Autodesk Fusion 360 part; units mm, degrees
(part 5 of 7)
  spline S20 degree 5 poles (-19.6631, 0.6054) (-19.6646, 0.6091) (-19.6677, 0.6165) (-19.6726, 0.6274) (-19.6799, 0.6416) (-19.6898, 0.659) (-19.7004, 0.6761) (-19.7114, 0.6931) (-19.7226, 0.7099) (-19.734, 0.7267) (-19.7456, 0.7434) (-19.7573, 0.76) (-19.7694, 0.7765) (-19.7817, 0.7928) (-19.7944, 0.809) (-19.8073, 0.825) (-19.8205, 0.8409) (-19.834, 0.8567) (-19.8476, 0.8724) (-19.8613, 0.888) (-19.8753, 0.9035) (-19.8895, 0.919) (-19.9038, 0.9343) (-19.9183, 0.9495) (-19.9331, 0.9646) (-19.948, 0.9796) (-19.9631, 0.9945) (-19.9784, 1.0092) (-19.9938, 1.0239) (-20.0094, 1.0385) (-20.0251, 1.0531) (-20.0411, 1.0675) (-20.0571, 1.0818) (-20.0734, 1.096) (-20.0898, 1.1101) (-20.1063, 1.1242) (-20.123, 1.1381) (-20.1398, 1.1519) (-20.1568, 1.1657) (-20.174, 1.1793) (-20.1912, 1.1929) (-20.2087, 1.2063) (-20.2262, 1.2197) (-20.2439, 1.233) (-20.2617, 1.2461) (-20.2797, 1.2592) (-20.2978, 1.2722) (-20.316, 1.2851) (-20.3344, 1.2979) (-20.3529, 1.3106) (-20.3715, 1.3232) (-20.3902, 1.3357) (-20.4091, 1.3481) (-20.4281, 1.3604) (-20.4472, 1.3727) (-20.4664, 1.3848) (-20.4858, 1.3968) (-20.5053, 1.4088) (-20.5249, 1.4206) (-20.5446, 1.4323) (-20.5644, 1.444) (-20.5844, 1.4556) (-20.6044, 1.467) (-20.6246, 1.4784) (-20.6449, 1.4896) (-20.6653, 1.5008) (-20.6858, 1.5119) (-20.7064, 1.5228) (-20.7272, 1.5337) (-20.748, 1.5445) (-20.7689, 1.5552) (-20.7858, 1.5636) (-20.7985, 1.5699) (-20.8069, 1.5741) (-20.8112, 1.5762) knots 0 0 0 0 0 0 0.01428571 0.02857143 0.04285714 0.05714286 0.07142857 0.08571429 0.1 0.11428571 0.12857143 0.14285714 0.15714286 0.17142857 0.18571429 0.2 0.21428571 0.22857143 0.24285714 0.25714286 0.27142857 0.28571429 0.3 0.31428571 0.32857143 0.34285714 0.35714286 0.37142857 0.38571429 0.4 0.41428571 0.42857143 0.44285714 0.45714286 0.47142857 0.48571429 0.5 0.51428571 0.52857143 0.54285714 0.55714286 0.57142857 0.58571429 0.6 0.61428571 0.62857143 0.64285714 0.65714286 0.67142857 0.68571429 0.7 0.71428571 0.72857143 0.74285714 0.75714286 0.77142857 0.78571429 0.8 0.81428571 0.82857143 0.84285714 0.85714286 0.87142857 0.88571429 0.9 0.91428571 0.92857143 0.94285714 0.95714286 0.97142857 0.98571429 1 1 1 1 1 1
  arc A21 (-20.8112, 1.5762) -> (-21.3487, 1.2659) centre (-17.5834, -4.6352) ccw
  spline S21 degree 5 poles (-21.3487, 1.2659) (-21.349, 1.2612) (-21.3496, 1.2517) (-21.3505, 1.2376) (-21.3516, 1.2188) (-21.3528, 1.1953) (-21.3539, 1.1719) (-21.3549, 1.1485) (-21.3557, 1.1251) (-21.3563, 1.1018) (-21.3569, 1.0786) (-21.3573, 1.0554) (-21.3575, 1.0322) (-21.3576, 1.0091) (-21.3576, 0.9861) (-21.3574, 0.9631) (-21.3571, 0.9401) (-21.3566, 0.9172) (-21.356, 0.8944) (-21.3553, 0.8716) (-21.3544, 0.8489) (-21.3534, 0.8262) (-21.3522, 0.8036) (-21.3509, 0.7811) (-21.3494, 0.7586) (-21.3478, 0.7361) (-21.3461, 0.7138) (-21.3442, 0.6915) (-21.3421, 0.6693) (-21.3399, 0.6471) (-21.3376, 0.625) (-21.3351, 0.603) (-21.3324, 0.581) (-21.3296, 0.5591) (-21.3267, 0.5373) (-21.3236, 0.5156) (-21.3203, 0.4939) (-21.3169, 0.4723) (-21.3134, 0.4508) (-21.3096, 0.4294) (-21.3058, 0.4081) (-21.3017, 0.3868) (-21.2975, 0.3656) (-21.2932, 0.3446) (-21.2887, 0.3236) (-21.284, 0.3027) (-21.2791, 0.2819) (-21.2741, 0.2611) (-21.2689, 0.2405) (-21.2636, 0.22) (-21.2581, 0.1996) (-21.2524, 0.1793) (-21.2465, 0.1591) (-21.2404, 0.139) (-21.2341, 0.119) (-21.2276, 0.0992) (-21.221, 0.0795) (-21.2142, 0.0598) (-21.2072, 0.0403) (-21.2001, 0.0209) (-21.1927, 0.0017) (-21.185, -0.0174) (-21.177, -0.0362) (-21.1688, -0.0549) (-21.1603, -0.0734) (-21.1516, -0.0917) (-21.1427, -0.11) (-21.1338, -0.1281) (-21.1246, -0.1461) (-21.1151, -0.1638) (-21.105, -0.1811) (-21.0963, -0.1945) (-21.0893, -0.2043) (-21.0844, -0.2106) (-21.082, -0.2138) knots -1 -1 -1 -1 -1 -1 -0.98571429 -0.97142857 -0.95714286 -0.94285714 -0.92857143 -0.91428571 -0.9 -0.88571429 -0.87142857 -0.85714286 -0.84285714 -0.82857143 -0.81428571 -0.8 -0.78571429 -0.77142857 -0.75714286 -0.74285714 -0.72857143 -0.71428571 -0.7 -0.68571429 -0.67142857 -0.65714286 -0.64285714 -0.62857143 -0.61428571 -0.6 -0.58571429 -0.57142857 -0.55714286 -0.54285714 -0.52857143 -0.51428571 -0.5 -0.48571429 -0.47142857 -0.45714286 -0.44285714 -0.42857143 -0.41428571 -0.4 -0.38571429 -0.37142857 -0.35714286 -0.34285714 -0.32857143 -0.31428571 -0.3 -0.28571429 -0.27142857 -0.25714286 -0.24285714 -0.22857143 -0.21428571 -0.2 -0.18571429 -0.17142857 -0.15714286 -0.14285714 -0.12857143 -0.11428571 -0.1 -0.08571429 -0.07142857 -0.05714286 -0.04285714 -0.02857143 -0.01428571 0 0 0 0 0 0
  line L21 (-21.082, -0.2138) -> (-20.5315, -0.9118)
  arc A22 (-20.5315, -0.9118) -> (-21.3068, -1.6871) centre (-17.5834, -4.6352) ccw
  line L22 (-21.3068, -1.6871) -> (-22.0048, -1.1366)
  spline S22 degree 5 poles (-22.0048, -1.1366) (-22.0079, -1.1341) (-22.0143, -1.1293) (-22.024, -1.1223) (-22.0374, -1.1136) (-22.0547, -1.1035) (-22.0724, -1.094) (-22.0904, -1.0848) (-22.1086, -1.0758) (-22.1268, -1.067) (-22.1452, -1.0583) (-22.1637, -1.0498) (-22.1823, -1.0415) (-22.2012, -1.0336) (-22.2202, -1.0259) (-22.2395, -1.0185) (-22.2589, -1.0113) (-22.2784, -1.0043) (-22.298, -0.9976) (-22.3178, -0.9909) (-22.3376, -0.9845) (-22.3576, -0.9782) (-22.3776, -0.9721) (-22.3978, -0.9662) (-22.4181, -0.9605) (-22.4386, -0.955) (-22.4591, -0.9496) (-22.4797, -0.9444) (-22.5004, -0.9394) (-22.5212, -0.9346) (-22.5421, -0.9299) (-22.5631, -0.9254) (-22.5842, -0.921) (-22.6054, -0.9168) (-22.6266, -0.9128) (-22.648, -0.9089) (-22.6694, -0.9052) (-22.6909, -0.9016) (-22.7125, -0.8982) (-22.7341, -0.895) (-22.7559, -0.8919) (-22.7777, -0.8889) (-22.7996, -0.8861) (-22.8215, -0.8835) (-22.8436, -0.881) (-22.8657, -0.8786) (-22.8878, -0.8765) (-22.91, -0.8744) (-22.9323, -0.8725) (-22.9547, -0.8707) (-22.9771, -0.8691) (-22.9996, -0.8677) (-23.0222, -0.8664) (-23.0448, -0.8652) (-23.0674, -0.8642) (-23.0902, -0.8633) (-23.113, -0.8625) (-23.1358, -0.8619) (-23.1587, -0.8615) (-23.1816, -0.8612) (-23.2046, -0.861) (-23.2277, -0.8609) (-23.2508, -0.8611) (-23.2739, -0.8613) (-23.2971, -0.8617) (-23.3204, -0.8622) (-23.3437, -0.8629) (-23.367, -0.8637) (-23.3904, -0.8646) (-23.4139, -0.8657) (-23.4373, -0.867) (-23.4561, -0.868) (-23.4703, -0.8689) (-23.4797, -0.8695) (-23.4844, -0.8698) knots 0 0 0 0 0 0 0.01428571 0.02857143 0.04285714 0.05714286 0.07142857 0.08571429 0.1 0.11428571 0.12857143 0.14285714 0.15714286 0.17142857 0.18571429 0.2 0.21428571 0.22857143 0.24285714 0.25714286 0.27142857 0.28571429 0.3 0.31428571 0.32857143 0.34285714 0.35714286 0.37142857 0.38571429 0.4 0.41428571 0.42857143 0.44285714 0.45714286 0.47142857 0.48571429 0.5 0.51428571 0.52857143 0.54285714 0.55714286 0.57142857 0.58571429 0.6 0.61428571 0.62857143 0.64285714 0.65714286 0.67142857 0.68571429 0.7 0.71428571 0.72857143 0.74285714 0.75714286 0.77142857 0.78571429 0.8 0.81428571 0.82857143 0.84285714 0.85714286 0.87142857 0.88571429 0.9 0.91428571 0.92857143 0.94285714 0.95714286 0.97142857 0.98571429 1 1 1 1 1 1
  arc A23 (-23.4844, -0.8698) -> (-23.7948, -1.4074) centre (-17.5834, -4.6352) ccw
  spline S23 degree 5 poles (-23.7948, -1.4074) (-23.7927, -1.4116) (-23.7885, -1.4201) (-23.7822, -1.4328) (-23.7737, -1.4496) (-23.7631, -1.4706) (-23.7523, -1.4914) (-23.7414, -1.5121) (-23.7304, -1.5327) (-23.7194, -1.5533) (-23.7082, -1.5737) (-23.6969, -1.5939) (-23.6856, -1.6141) (-23.6741, -1.6342) (-23.6626, -1.6541) (-23.6509, -1.674) (-23.6392, -1.6937) (-23.6273, -1.7133) (-23.6154, -1.7328) (-23.6033, -1.7521) (-23.5912, -1.7713) (-23.579, -1.7905) (-23.5667, -1.8095) (-23.5543, -1.8283) (-23.5417, -1.8471) (-23.5291, -1.8657) (-23.5164, -1.8842) (-23.5036, -1.9025) (-23.4907, -1.9208) (-23.4778, -1.9389) (-23.4647, -1.9568) (-23.4515, -1.9747) (-23.4382, -1.9923) (-23.4249, -2.0099) (-23.4114, -2.0273) (-23.3979, -2.0446) (-23.3842, -2.0617) (-23.3705, -2.0787) (-23.3566, -2.0956) (-23.3427, -2.1122) (-23.3287, -2.1288) (-23.3146, -2.1452) (-23.3003, -2.1614) (-23.286, -2.1775) (-23.2716, -2.1934) (-23.2571, -2.2092) (-23.2425, -2.2248) (-23.2278, -2.2402) (-23.213, -2.2555) (-23.1981, -2.2706) (-23.1831, -2.2855) (-23.168, -2.3002) (-23.1528, -2.3148) (-23.1375, -2.3291) (-23.1221, -2.3432) (-23.1066, -2.3572) (-23.091, -2.371) (-23.0753, -2.3846) (-23.0595, -2.398) (-23.0436, -2.4112) (-23.0275, -2.4242) (-23.0114, -2.4368) (-22.995, -2.4492) (-22.9786, -2.4612) (-22.9619, -2.473) (-22.9452, -2.4845) (-22.9285, -2.4959) (-22.9116, -2.5071) (-22.8947, -2.5181) (-22.8776, -2.5287) (-22.8602, -2.5387) (-22.8459, -2.5459) (-22.835, -2.5509) (-22.8277, -2.5539) (-22.8239, -2.5554) knots -1 -1 -1 -1 -1 -1 -0.98571429 -0.97142857 -0.95714286 -0.94285714 -0.92857143 -0.91428571 -0.9 -0.88571429 -0.87142857 -0.85714286 -0.84285714 -0.82857143 -0.81428571 -0.8 -0.78571429 -0.77142857 -0.75714286 -0.74285714 -0.72857143 -0.71428571 -0.7 -0.68571429 -0.67142857 -0.65714286 -0.64285714 -0.62857143 -0.61428571 -0.6 -0.58571429 -0.57142857 -0.55714286 -0.54285714 -0.52857143 -0.51428571 -0.5 -0.48571429 -0.47142857 -0.45714286 -0.44285714 -0.42857143 -0.41428571 -0.4 -0.38571429 -0.37142857 -0.35714286 -0.34285714 -0.32857143 -0.31428571 -0.3 -0.28571429 -0.27142857 -0.25714286 -0.24285714 -0.22857143 -0.21428571 -0.2 -0.18571429 -0.17142857 -0.15714286 -0.14285714 -0.12857143 -0.11428571 -0.1 -0.08571429 -0.07142857 -0.05714286 -0.04285714 -0.02857143 -0.01428571 0 0 0 0 0 0
  line L23 (-22.8239, -2.5554) -> (-21.9982, -2.8847)
  circle A24 centre (-17.5834, -4.6352) radius 2.5
  dimension "d37" = 5
  constraint concentric A0 A24
  measures "d37" diameter of A24
extrude "Extrude3'" add sketch "Sketch3 (5)" along normal blind 70 contours A24 sketch seen with x (1, 0, 0) y (0, 1, 0) z (0, 0, 1) at (-17.5834, -4.6352, 11.1752) bodies 2 in component "Spur Gear (12 teeth) (1)"
sketch "Sketch4" plane through (0, 0, 10) normal (0, 0, 1) x (-1, 0, 0)
  line L0 (-2.75, -1.85) -> (-2.75, 1.85)
  line L1 (-2.75, 1.85) -> (2.75, 1.85)
  line L2 (2.75, 1.85) -> (2.75, -1.85)
  line L3 (2.75, -1.85) -> (-2.75, -1.85)
  arc A0 (-10.5729, 1.9389) -> (-10.7145, 0.8636) centre (0, 0) ccw
  line L4 (-10.7145, 0.8636) -> (-11.2399, 0.9051)
  spline S0 degree 5 poles (-11.2399, 0.9051) (-11.2449, 0.9055) (-11.255, 0.9062) (-11.27, 0.9068) (-11.2901, 0.907) (-11.3152, 0.9062) (-11.3404, 0.9047) (-11.3655, 0.9028) (-11.3907, 0.9006) (-11.416, 0.8982) (-11.4412, 0.8957) (-11.4664, 0.8929) (-11.4917, 0.8899) (-11.5169, 0.8866) (-11.5422, 0.8828) (-11.5674, 0.8788) (-11.5927, 0.8745) (-11.6179, 0.87) (-11.6432, 0.8652) (-11.6685, 0.8603) (-11.6937, 0.8552) (-11.719, 0.8499) (-11.7443, 0.8443) (-11.7695, 0.8386) (-11.7948, 0.8327) (-11.82, 0.8265) (-11.8453, 0.8202) (-11.8706, 0.8136) (-11.8958, 0.8069) (-11.921, 0.8) (-11.9463, 0.7929) (-11.9715, 0.7857) (-11.9967, 0.7783) (-12.0219, 0.7707) (-12.0471, 0.7629) (-12.0723, 0.755) (-12.0975, 0.7469) (-12.1227, 0.7387) (-12.1479, 0.7302) (-12.173, 0.7217) (-12.1982, 0.7129) (-12.2233, 0.7041) (-12.2484, 0.695) (-12.2735, 0.6858) (-12.2986, 0.6765) (-12.3237, 0.667) (-12.3488, 0.6573) (-12.3739, 0.6475) (-12.3989, 0.6376) (-12.424, 0.6275) (-12.449, 0.6173) (-12.474, 0.6069) (-12.499, 0.5964) (-12.5239, 0.5858) (-12.5489, 0.575) (-12.5738, 0.564) (-12.5988, 0.553) (-12.6237, 0.5418) (-12.6486, 0.5304) (-12.6735, 0.5189) (-12.6983, 0.5073) (-12.7232, 0.4956) (-12.748, 0.4837) (-12.7728, 0.4717) (-12.7976, 0.4595) (-12.8223, 0.4473) (-12.8471, 0.4349) (-12.8718, 0.4223) (-12.8965, 0.4097) (-12.9212, 0.3969) (-12.9458, 0.384) (-12.9655, 0.3735) (-12.9803, 0.3657) (-12.9902, 0.3604) (-12.9951, 0.3577) knots 0 0 0 0 0 0 0.01428571 0.02857143 0.04285714 0.05714286 0.07142857 0.08571429 0.1 0.11428571 0.12857143 0.14285714 0.15714286 0.17142857 0.18571429 0.2 0.21428571 0.22857143 0.24285714 0.25714286 0.27142857 0.28571429 0.3 0.31428571 0.32857143 0.34285714 0.35714286 0.37142857 0.38571429 0.4 0.41428571 0.42857143 0.44285714 0.45714286 0.47142857 0.48571429 0.5 0.51428571 0.52857143 0.54285714 0.55714286 0.57142857 0.58571429 0.6 0.61428571 0.62857143 0.64285714 0.65714286 0.67142857 0.68571429 0.7 0.71428571 0.72857143 0.74285714 0.75714286 0.77142857 0.78571429 0.8 0.81428571 0.82857143 0.84285714 0.85714286 0.87142857 0.88571429 0.9 0.91428571 0.92857143 0.94285714 0.95714286 0.97142857 0.98571429 1 1 1 1 1 1
  arc A1 (-12.9951, 0.3577) -> (-12.9951, -0.3577) centre (0, 0) ccw
  spline S1 degree 5 poles (-12.9951, -0.3577) (-12.9902, -0.3604) (-12.9803, -0.3657) (-12.9655, -0.3735) (-12.9458, -0.384) (-12.9212, -0.3969) (-12.8965, -0.4097) (-12.8718, -0.4223) (-12.8471, -0.4349) (-12.8223, -0.4473) (-12.7976, -0.4595) (-12.7728, -0.4717) (-12.748, -0.4837) (-12.7232, -0.4956) (-12.6983, -0.5073) (-12.6735, -0.5189) (-12.6486, -0.5304) (-12.6237, -0.5418) (-12.5988, -0.553) (-12.5738, -0.564) (-12.5489, -0.575) (-12.5239, -0.5858) (-12.499, -0.5964) (-12.474, -0.6069) (-12.449, -0.6173) (-12.424, -0.6275) (-12.3989, -0.6376) (-12.3739, -0.6475) (-12.3488, -0.6573) (-12.3237, -0.667) (-12.2986, -0.6765) (-12.2735, -0.6858) (-12.2484, -0.695) (-12.2233, -0.7041) (-12.1982, -0.7129) (-12.173, -0.7217) (-12.1479, -0.7302) (-12.1227, -0.7387) (-12.0975, -0.7469) (-12.0723, -0.755) (-12.0471, -0.7629) (-12.0219, -0.7707) (-11.9967, -0.7783) (-11.9715, -0.7857) (-11.9463, -0.7929) (-11.921, -0.8) (-11.8958, -0.8069) (-11.8706, -0.8136) (-11.8453, -0.8202) (-11.82, -0.8265) (-11.7948, -0.8327) (-11.7695, -0.8386) (-11.7443, -0.8443) (-11.719, -0.8499) (-11.6937, -0.8552) (-11.6685, -0.8603) (-11.6432, -0.8652) (-11.6179, -0.87) (-11.5927, -0.8745) (-11.5674, -0.8788) (-11.5422, -0.8828) (-11.5169, -0.8866) (-11.4917, -0.8899) (-11.4664, -0.8929) (-11.4412, -0.8957) (-11.416, -0.8982) (-11.3907, -0.9006) (-11.3655, -0.9028) (-11.3404, -0.9047) (-11.3152, -0.9062) (-11.2901, -0.907) (-11.27, -0.9068) (-11.255, -0.9062) (-11.2449, -0.9055) (-11.2399, -0.9051) knots -1 -1 -1 -1 -1 -1 -0.98571429 -0.97142857 -0.95714286 -0.94285714 -0.92857143 -0.91428571 -0.9 -0.88571429 -0.87142857 -0.85714286 -0.84285714 -0.82857143 -0.81428571 -0.8 -0.78571429 -0.77142857 -0.75714286 -0.74285714 -0.72857143 -0.71428571 -0.7 -0.68571429 -0.67142857 -0.65714286 -0.64285714 -0.62857143 -0.61428571 -0.6 -0.58571429 -0.57142857 -0.55714286 -0.54285714 -0.52857143 -0.51428571 -0.5 -0.48571429 -0.47142857 -0.45714286 -0.44285714 -0.42857143 -0.41428571 -0.4 -0.38571429 -0.37142857 -0.35714286 -0.34285714 -0.32857143 -0.31428571 -0.3 -0.28571429 -0.27142857 -0.25714286 -0.24285714 -0.22857143 -0.21428571 -0.2 -0.18571429 -0.17142857 -0.15714286 -0.14285714 -0.12857143 -0.11428571 -0.1 -0.08571429 -0.07142857 -0.05714286 -0.04285714 -0.02857143 -0.01428571 0 0 0 0 0 0
  line L5 (-11.2399, -0.9051) -> (-10.7145, -0.8636)
  arc A2 (-10.7145, -0.8636) -> (-10.5729, -1.9389) centre (0, 0) ccw
  line L6 (-10.5729, -1.9389) -> (-11.0912, -2.0348)
  spline S2 degree 5 poles (-11.0912, -2.0348) (-11.0961, -2.0357) (-11.106, -2.0377) (-11.1207, -2.041) (-11.1401, -2.046) (-11.1642, -2.0533) (-11.1881, -2.0612) (-11.2119, -2.0696) (-11.2357, -2.0783) (-11.2594, -2.0871) (-11.2831, -2.096) (-11.3068, -2.1052) (-11.3304, -2.1147) (-11.3539, -2.1244) (-11.3774, -2.1346) (-11.4007, -2.145) (-11.424, -2.1557) (-11.4472, -2.1666) (-11.4704, -2.1777) (-11.4935, -2.189) (-11.5166, -2.2005) (-11.5397, -2.2122) (-11.5626, -2.2241) (-11.5855, -2.2361) (-11.6084, -2.2484) (-11.6312, -2.2609) (-11.654, -2.2736) (-11.6767, -2.2864) (-11.6993, -2.2995) (-11.7219, -2.3126) (-11.7444, -2.326) (-11.7669, -2.3395) (-11.7894, -2.3532) (-11.8118, -2.3671) (-11.8341, -2.3811) (-11.8564, -2.3953) (-11.8786, -2.4096) (-11.9008, -2.4241) (-11.9229, -2.4387) (-11.945, -2.4535) (-11.967, -2.4685) (-11.989, -2.4836) (-12.011, -2.4988) (-12.0328, -2.5142) (-12.0547, -2.5297) (-12.0764, -2.5454) (-12.0982, -2.5612) (-12.1198, -2.5771) (-12.1415, -2.5932) (-12.163, -2.6094) (-12.1846, -2.6258) (-12.206, -2.6423) (-12.2274, -2.6589) (-12.2488, -2.6756) (-12.2701, -2.6925) (-12.2914, -2.7095) (-12.3126, -2.7267) (-12.3338, -2.744) (-12.3549, -2.7614) (-12.3759, -2.7789) (-12.3969, -2.7965) (-12.4179, -2.8143) (-12.4388, -2.8322) (-12.4596, -2.8502) (-12.4804, -2.8684) (-12.5012, -2.8866) (-12.5219, -2.905) (-12.5425, -2.9235) (-12.5631, -2.9421) (-12.5836, -2.9609) (-12.6041, -2.9797) (-12.6204, -2.9949) (-12.6327, -3.0064) (-12.6408, -3.014) (-12.6449, -3.0178) knots 0 0 0 0 0 0 0.01428571 0.02857143 0.04285714 0.05714286 0.07142857 0.08571429 0.1 0.11428571 0.12857143 0.14285714 0.15714286 0.17142857 0.18571429 0.2 0.21428571 0.22857143 0.24285714 0.25714286 0.27142857 0.28571429 0.3 0.31428571 0.32857143 0.34285714 0.35714286 0.37142857 0.38571429 0.4 0.41428571 0.42857143 0.44285714 0.45714286 0.47142857 0.48571429 0.5 0.51428571 0.52857143 0.54285714 0.55714286 0.57142857 0.58571429 0.6 0.61428571 0.62857143 0.64285714 0.65714286 0.67142857 0.68571429 0.7 0.71428571 0.72857143 0.74285714 0.75714286 0.77142857 0.78571429 0.8 0.81428571 0.82857143 0.84285714 0.85714286 0.87142857 0.88571429 0.9 0.91428571 0.92857143 0.94285714 0.95714286 0.97142857 0.98571429 1 1 1 1 1 1
  arc A3 (-12.6449, -3.0178) -> (-12.4597, -3.7089) centre (0, 0) ccw
  spline S3 degree 5 poles (-12.4597, -3.7089) (-12.4543, -3.7102) (-12.4434, -3.7127) (-12.4271, -3.7165) (-12.4053, -3.7215) (-12.3782, -3.7276) (-12.351, -3.7336) (-12.3239, -3.7394) (-12.2968, -3.7451) (-12.2696, -3.7507) (-12.2426, -3.7561) (-12.2155, -3.7614) (-12.1884, -3.7666) (-12.1614, -3.7717) (-12.1343, -3.7766) (-12.1073, -3.7814) (-12.0803, -3.786) (-12.0533, -3.7905) (-12.0264, -3.7949) (-11.9994, -3.7992) (-11.9725, -3.8033) (-11.9456, -3.8072) (-11.9187, -3.8111) (-11.8919, -3.8147) (-11.865, -3.8183) (-11.8382, -3.8217) (-11.8114, -3.825) (-11.7846, -3.8281) (-11.7579, -3.831) (-11.7312, -3.8339) (-11.7045, -3.8365) (-11.6778, -3.8391) (-11.6512, -3.8415) (-11.6246, -3.8437) (-11.598, -3.8458) (-11.5714, -3.8477) (-11.5449, -3.8495) (-11.5184, -3.8511) (-11.492, -3.8525) (-11.4656, -3.8538) (-11.4392, -3.855) (-11.4128, -3.8559) (-11.3865, -3.8567) (-11.3602, -3.8574) (-11.334, -3.8578) (-11.3078, -3.8581) (-11.2816, -3.8583) (-11.2555, -3.8582) (-11.2294, -3.858) (-11.2034, -3.8576) (-11.1774, -3.857) (-11.1514, -3.8562) (-11.1256, -3.8552) (-11.0997, -3.854) (-11.0739, -3.8526) (-11.0482, -3.851) (-11.0225, -3.8492) (-10.9969, -3.8473) (-10.9713, -3.8451) (-10.9458, -3.8427) (-10.9204, -3.8401) (-10.895, -3.8371) (-10.8698, -3.8339) (-10.8446, -3.8302) (-10.8195, -3.8264) (-10.7945, -3.8223) (-10.7695, -3.818) (-10.7446, -3.8136) (-10.7198, -3.809) (-10.6951, -3.8039) (-10.6706, -3.7981) (-10.6513, -3.7928) (-10.6369, -3.7883) (-10.6274, -3.7851) (-10.6227, -3.7834) knots -1 -1 -1 -1 -1 -1 -0.98571429 -0.97142857 -0.95714286 -0.94285714 -0.92857143 -0.91428571 -0.9 -0.88571429 -0.87142857 -0.85714286 -0.84285714 -0.82857143 -0.81428571 -0.8 -0.78571429 -0.77142857 -0.75714286 -0.74285714 -0.72857143 -0.71428571 -0.7 -0.68571429 -0.67142857 -0.65714286 -0.64285714 -0.62857143 -0.61428571 -0.6 -0.58571429 -0.57142857 -0.55714286 -0.54285714 -0.52857143 -0.51428571 -0.5 -0.48571429 -0.47142857 -0.45714286 -0.44285714 -0.42857143 -0.41428571 -0.4 -0.38571429 -0.37142857 -0.35714286 -0.34285714 -0.32857143 -0.31428571 -0.3 -0.28571429 -0.27142857 -0.25714286 -0.24285714 -0.22857143 -0.21428571 -0.2 -0.18571429 -0.17142857 -0.15714286 -0.14285714 -0.12857143 -0.11428571 -0.1 -0.08571429 -0.07142857 -0.05714286 -0.04285714 -0.02857143 -0.01428571 0 0 0 0 0 0
  line L7 (-10.6227, -3.7834) -> (-10.1259, -3.6073)
  arc A4 (-10.1259, -3.6073) -> (-9.7108, -4.6093) centre (0, 0) ccw
  line L8 (-9.7108, -4.6093) -> (-10.1866, -4.8361)
  spline S4 degree 5 poles (-10.1866, -4.8361) (-10.1912, -4.8383) (-10.2002, -4.8427) (-10.2135, -4.8497) (-10.231, -4.8596) (-10.2523, -4.8728) (-10.2734, -4.8867) (-10.2942, -4.901) (-10.315, -4.9155) (-10.3356, -4.9301) (-10.3562, -4.9449) (-10.3767, -4.9599) (-10.397, -4.9751) (-10.4172, -4.9907) (-10.4372, -5.0065) (-10.4571, -5.0226) (-10.4768, -5.039) (-10.4964, -5.0555) (-10.5159, -5.0723) (-10.5353, -5.0892) (-10.5547, -5.1063) (-10.5739, -5.1235) (-10.593, -5.1409) (-10.612, -5.1585) (-10.6309, -5.1763) (-10.6497, -5.1942) (-10.6684, -5.2124) (-10.687, -5.2307) (-10.7055, -5.2491) (-10.7239, -5.2677) (-10.7422, -5.2864) (-10.7605, -5.3053) (-10.7786, -5.3243) (-10.7966, -5.3435) (-10.8146, -5.3628) (-10.8324, -5.3823) (-10.8502, -5.4019) (-10.8679, -5.4216) (-10.8855, -5.4415) (-10.903, -5.4615) (-10.9204, -5.4817) (-10.9377, -5.5019) (-10.955, -5.5223) (-10.9721, -5.5428) (-10.9892, -5.5635) (-11.0062, -5.5842) (-11.023, -5.6051) (-11.0399, -5.6261) (-11.0566, -5.6473) (-11.0732, -5.6685) (-11.0898, -5.6899) (-11.1062, -5.7114) (-11.1226, -5.733) (-11.1389, -5.7547) (-11.1552, -5.7765) (-11.1713, -5.7985) (-11.1873, -5.8205) (-11.2033, -5.8427) (-11.2192, -5.8649) (-11.235, -5.8873) (-11.2507, -5.9098) (-11.2664, -5.9324) (-11.2819, -5.9551) (-11.2974, -5.9779) (-11.3128, -6.0008) (-11.3281, -6.0238) (-11.3433, -6.0469) (-11.3585, -6.0701) (-11.3735, -6.0935) (-11.3885, -6.1169) (-11.4034, -6.1404) (-11.4153, -6.1593) (-11.4241, -6.1735) (-11.43, -6.183) (-11.4329, -6.1877) knots 0 0 0 0 0 0 0.01428571 0.02857143 0.04285714 0.05714286 0.07142857 0.08571429 0.1 0.11428571 0.12857143 0.14285714 0.15714286 0.17142857 0.18571429 0.2 0.21428571 0.22857143 0.24285714 0.25714286 0.27142857 0.28571429 0.3 0.31428571 0.32857143 0.34285714 0.35714286 0.37142857 0.38571429 0.4 0.41428571 0.42857143 0.44285714 0.45714286 0.47142857 0.48571429 0.5 0.51428571 0.52857143 0.54285714 0.55714286 0.57142857 0.58571429 0.6 0.61428571 0.62857143 0.64285714 0.65714286 0.67142857 0.68571429 0.7 0.71428571 0.72857143 0.74285714 0.75714286 0.77142857 0.78571429 0.8 0.81428571 0.82857143 0.84285714 0.85714286 0.87142857 0.88571429 0.9 0.91428571 0.92857143 0.94285714 0.95714286 0.97142857 0.98571429 1 1 1 1 1 1
  arc A5 (-11.4329, -6.1877) -> (-11.0752, -6.8073) centre (0, 0) ccw
  spline S5 degree 5 poles (-11.0752, -6.8073) (-11.0696, -6.8072) (-11.0585, -6.8068) (-11.0417, -6.8063) (-11.0194, -6.8054) (-10.9916, -6.8043) (-10.9638, -6.803) (-10.9361, -6.8016) (-10.9085, -6.8001) (-10.8808, -6.7985) (-10.8532, -6.7967) (-10.8257, -6.7949) (-10.7982, -6.7929) (-10.7708, -6.7908) (-10.7434, -6.7885) (-10.7161, -6.7861) (-10.6888, -6.7836) (-10.6616, -6.781) (-10.6344, -6.7783) (-10.6073, -6.7754) (-10.5802, -6.7724) (-10.5532, -6.7693) (-10.5262, -6.766) (-10.4993, -6.7626) (-10.4725, -6.7591) (-10.4457, -6.7554) (-10.419, -6.7516) (-10.3923, -6.7477) (-10.3657, -6.7437) (-10.3392, -6.7395) (-10.3127, -6.7352) (-10.2863, -6.7307) (-10.2599, -6.7261) (-10.2337, -6.7214) (-10.2074, -6.7165) (-10.1813, -6.7115) (-10.1552, -6.7063) (-10.1292, -6.701) (-10.1033, -6.6956) (-10.0774, -6.69) (-10.0516, -6.6843) (-10.0259, -6.6784) (-10.0003, -6.6724) (-9.9748, -6.6662) (-9.9493, -6.6598) (-9.9239, -6.6533) (-9.8986, -6.6467) (-9.8734, -6.6399) (-9.8483, -6.6329) (-9.8232, -6.6258) (-9.7983, -6.6185) (-9.7734, -6.611) (-9.7487, -6.6034) (-9.724, -6.5955) (-9.6995, -6.5875) (-9.675, -6.5793) (-9.6507, -6.5709) (-9.6264, -6.5624) (-9.6023, -6.5537) (-9.5783, -6.5448) (-9.5544, -6.5356) (-9.5307, -6.5262) (-9.5071, -6.5165) (-9.4837, -6.5065) (-9.4605, -6.4963) (-9.4374, -6.4859) (-9.4144, -6.4753) (-9.3915, -6.4646) (-9.3687, -6.4537) (-9.3462, -6.4424) (-9.324, -6.4305) (-9.3067, -6.4203) (-9.294, -6.4123) (-9.2856, -6.4067) (-9.2815, -6.4038) knots -1 -1 -1 -1 -1 -1 -0.98571429 -0.97142857 -0.95714286 -0.94285714 -0.92857143 -0.91428571 -0.9 -0.88571429 -0.87142857 -0.85714286 -0.84285714 -0.82857143 -0.81428571 -0.8 -0.78571429 -0.77142857 -0.75714286 -0.74285714 -0.72857143 -0.71428571 -0.7 -0.68571429 -0.67142857 -0.65714286 -0.64285714 -0.62857143 -0.61428571 -0.6 -0.58571429 -0.57142857 -0.55714286 -0.54285714 -0.52857143 -0.51428571 -0.5 -0.48571429 -0.47142857 -0.45714286 -0.44285714 -0.42857143 -0.41428571 -0.4 -0.38571429 -0.37142857 -0.35714286 -0.34285714 -0.32857143 -0.31428571 -0.3 -0.28571429 -0.27142857 -0.25714286 -0.24285714 -0.22857143 -0.21428571 -0.2 -0.18571429 -0.17142857 -0.15714286 -0.14285714 -0.12857143 -0.11428571 -0.1 -0.08571429 -0.07142857 -0.05714286 -0.04285714 -0.02857143 -0.01428571 0 0 0 0 0 0
  line L9 (-9.2815, -6.4038) -> (-8.8472, -6.1051)
  arc A6 (-8.8472, -6.1051) -> (-8.1869, -6.9656) centre (0, 0) ccw
  line L10 (-8.1869, -6.9656) -> (-8.5878, -7.3078)
  spline S6 degree 5 poles (-8.5878, -7.3078) (-8.5917, -7.3111) (-8.5992, -7.3177) (-8.6103, -7.3279) (-8.6246, -7.342) (-8.6418, -7.3603) (-8.6586, -7.3791) (-8.675, -7.3983) (-8.6913, -7.4177) (-8.7074, -7.4372) (-8.7235, -7.4568) (-8.7394, -7.4766) (-8.7551, -7.4966) (-8.7706, -7.5168) (-8.7858, -7.5373) (-8.8008, -7.558) (-8.8156, -7.5789) (-8.8303, -7.6) (-8.8448, -7.6212) (-8.8592, -7.6425) (-8.8734, -7.664) (-8.8875, -7.6856) (-8.9015, -7.7074) (-8.9153, -7.7293) (-8.929, -7.7514) (-8.9425, -7.7736) (-8.9558, -7.796) (-8.9691, -7.8184) (-8.9822, -7.841) (-8.9951, -7.8638) (-9.008, -7.8866) (-9.0207, -7.9096) (-9.0333, -7.9326) (-9.0457, -7.9558) (-9.0581, -7.9791) (-9.0703, -8.0025) (-9.0824, -8.0261) (-9.0943, -8.0497) (-9.1062, -8.0735) (-9.1179, -8.0973) (-9.1295, -8.1213) (-9.141, -8.1453) (-9.1524, -8.1695) (-9.1637, -8.1938) (-9.1748, -8.2181) (-9.1858, -8.2426) (-9.1967, -8.2671) (-9.2075, -8.2918) (-9.2182, -8.3165) (-9.2288, -8.3413) (-9.2392, -8.3663) (-9.2496, -8.3913) (-9.2598, -8.4164) (-9.27, -8.4416) (-9.28, -8.4669) (-9.2899, -8.4922) (-9.2997, -8.5177) (-9.3094, -8.5432) (-9.319, -8.5688) (-9.3284, -8.5945) (-9.3378, -8.6203) (-9.347, -8.6462) (-9.3562, -8.6722) (-9.3652, -8.6982) (-9.3742, -8.7243) (-9.383, -8.7505) (-9.3917, -8.7768) (-9.4004, -8.8031) (-9.4089, -8.8295) (-9.4173, -8.856) (-9.4256, -8.8826) (-9.4321, -8.9039) (-9.437, -8.9199) (-9.4403, -8.9306) (-9.4419, -8.936) knots 0 0 0 0 0 0 0.01428571 0.02857143 0.04285714 0.05714286 0.07142857 0.08571429 0.1 0.11428571 0.12857143 0.14285714 0.15714286 0.17142857 0.18571429 0.2 0.21428571 0.22857143 0.24285714 0.25714286 0.27142857 0.28571429 0.3 0.31428571 0.32857143 0.34285714 0.35714286 0.37142857 0.38571429 0.4 0.41428571 0.42857143 0.44285714 0.45714286 0.47142857 0.48571429 0.5 0.51428571 0.52857143 0.54285714 0.55714286 0.57142857 0.58571429 0.6 0.61428571 0.62857143 0.64285714 0.65714286 0.67142857 0.68571429 0.7 0.71428571 0.72857143 0.74285714 0.75714286 0.77142857 0.78571429 0.8 0.81428571 0.82857143 0.84285714 0.85714286 0.87142857 0.88571429 0.9 0.91428571 0.92857143 0.94285714 0.95714286 0.97142857 0.98571429 1 1 1 1 1 1
  arc A7 (-9.4419, -8.936) -> (-8.936, -9.4419) centre (0, 0) ccw
  spline S7 degree 5 poles (-8.936, -9.4419) (-8.9306, -9.4403) (-8.9199, -9.437) (-8.9039, -9.4321) (-8.8826, -9.4256) (-8.856, -9.4173) (-8.8295, -9.4089) (-8.8031, -9.4004) (-8.7768, -9.3917) (-8.7505, -9.383) (-8.7243, -9.3742) (-8.6982, -9.3652) (-8.6722, -9.3562) (-8.6462, -9.347) (-8.6203, -9.3378) (-8.5945, -9.3284) (-8.5688, -9.319) (-8.5432, -9.3094) (-8.5177, -9.2997) (-8.4922, -9.2899) (-8.4669, -9.28) (-8.4416, -9.27) (-8.4164, -9.2598) (-8.3913, -9.2496) (-8.3663, -9.2392) (-8.3413, -9.2288) (-8.3165, -9.2182) (-8.2918, -9.2075) (-8.2671, -9.1967) (-8.2426, -9.1858) (-8.2181, -9.1748) (-8.1938, -9.1637) (-8.1695, -9.1524) (-8.1453, -9.141) (-8.1213, -9.1295) (-8.0973, -9.1179) (-8.0735, -9.1062) (-8.0497, -9.0943) (-8.0261, -9.0824) (-8.0025, -9.0703) (-7.9791, -9.0581) (-7.9558, -9.0457) (-7.9326, -9.0333) (-7.9096, -9.0207) (-7.8866, -9.008) (-7.8638, -8.9951) (-7.841, -8.9822) (-7.8184, -8.9691) (-7.796, -8.9558) (-7.7736, -8.9425) (-7.7514, -8.929) (-7.7293, -8.9153) (-7.7074, -8.9015) (-7.6856, -8.8875) (-7.664, -8.8734) (-7.6425, -8.8592) (-7.6212, -8.8448) (-7.6, -8.8303) (-7.5789, -8.8156) (-7.558, -8.8008) (-7.5373, -8.7858) (-7.5168, -8.7706) (-7.4966, -8.7551) (-7.4766, -8.7394) (-7.4568, -8.7235) (-7.4372, -8.7074) (-7.4177, -8.6913) (-7.3983, -8.675) (-7.3791, -8.6586) (-7.3603, -8.6418) (-7.342, -8.6246) (-7.3279, -8.6103) (-7.3177, -8.5992) (-7.3111, -8.5917) (-7.3078, -8.5878) knots -1 -1 -1 -1 -1 -1 -0.98571429 -0.97142857 -0.95714286 -0.94285714 -0.92857143 -0.91428571 -0.9 -0.88571429 -0.87142857 -0.85714286 -0.84285714 -0.82857143 -0.81428571 -0.8 -0.78571429 -0.77142857 -0.75714286 -0.74285714 -0.72857143 -0.71428571 -0.7 -0.68571429 -0.67142857 -0.65714286 -0.64285714 -0.62857143 -0.61428571 -0.6 -0.58571429 -0.57142857 -0.55714286 -0.54285714 -0.52857143 -0.51428571 -0.5 -0.48571429 -0.47142857 -0.45714286 -0.44285714 -0.42857143 -0.41428571 -0.4 -0.38571429 -0.37142857 -0.35714286 -0.34285714 -0.32857143 -0.31428571 -0.3 -0.28571429 -0.27142857 -0.25714286 -0.24285714 -0.22857143 -0.21428571 -0.2 -0.18571429 -0.17142857 -0.15714286 -0.14285714 -0.12857143 -0.11428571 -0.1 -0.08571429 -0.07142857 -0.05714286 -0.04285714 -0.02857143 -0.01428571 0 0 0 0 0 0
  line L11 (-7.3078, -8.5878) -> (-6.9656, -8.1869)
  arc A8 (-6.9656, -8.1869) -> (-6.1051, -8.8472) centre (0, 0) ccw
  line L12 (-6.1051, -8.8472) -> (-6.4038, -9.2815)
  spline S8 degree 5 poles (-6.4038, -9.2815) (-6.4067, -9.2856) (-6.4123, -9.294) (-6.4203, -9.3067) (-6.4305, -9.324) (-6.4424, -9.3462) (-6.4537, -9.3687) (-6.4646, -9.3915) (-6.4753, -9.4144) (-6.4859, -9.4374) (-6.4963, -9.4605) (-6.5065, -9.4837) (-6.5165, -9.5071) (-6.5262, -9.5307) (-6.5356, -9.5544) (-6.5448, -9.5783) (-6.5537, -9.6023) (-6.5624, -9.6264) (-6.5709, -9.6507) (-6.5793, -9.675) (-6.5875, -9.6995) (-6.5955, -9.724) (-6.6034, -9.7487) (-6.611, -9.7734) (-6.6185, -9.7983) (-6.6258, -9.8232) (-6.6329, -9.8483) (-6.6399, -9.8734) (-6.6467, -9.8986) (-6.6533, -9.9239) (-6.6598, -9.9493) (-6.6662, -9.9748) (-6.6724, -10.0003) (-6.6784, -10.0259) (-6.6843, -10.0516) (-6.69, -10.0774) (-6.6956, -10.1033) (-6.701, -10.1292) (-6.7063, -10.1552) (-6.7115, -10.1813) (-6.7165, -10.2074) (-6.7214, -10.2337) (-6.7261, -10.2599) (-6.7307, -10.2863) (-6.7352, -10.3127) (-6.7395, -10.3392) (-6.7437, -10.3657) (-6.7477, -10.3923) (-6.7516, -10.419) (-6.7554, -10.4457) (-6.7591, -10.4725) (-6.7626, -10.4993) (-6.766, -10.5262) (-6.7693, -10.5532) (-6.7724, -10.5802) (-6.7754, -10.6073) (-6.7783, -10.6344) (-6.781, -10.6616) (-6.7836, -10.6888) (-6.7861, -10.7161) (-6.7885, -10.7434) (-6.7908, -10.7708) (-6.7929, -10.7982) (-6.7949, -10.8257) (-6.7967, -10.8532) (-6.7985, -10.8808) (-6.8001, -10.9085) (-6.8016, -10.9361) (-6.803, -10.9638) (-6.8043, -10.9916) (-6.8054, -11.0194) (-6.8063, -11.0417) (-6.8068, -11.0585) (-6.8072, -11.0696) (-6.8073, -11.0752) knots 0 0 0 0 0 0 0.01428571 0.02857143 0.04285714 0.05714286 0.07142857 0.08571429 0.1 0.11428571 0.12857143 0.14285714 0.15714286 0.17142857 0.18571429 0.2 0.21428571 0.22857143 0.24285714 0.25714286 0.27142857 0.28571429 0.3 0.31428571 0.32857143 0.34285714 0.35714286 0.37142857 0.38571429 0.4 0.41428571 0.42857143 0.44285714 0.45714286 0.47142857 0.48571429 0.5 0.51428571 0.52857143 0.54285714 0.55714286 0.57142857 0.58571429 0.6 0.61428571 0.62857143 0.64285714 0.65714286 0.67142857 0.68571429 0.7 0.71428571 0.72857143 0.74285714 0.75714286 0.77142857 0.78571429 0.8 0.81428571 0.82857143 0.84285714 0.85714286 0.87142857 0.88571429 0.9 0.91428571 0.92857143 0.94285714 0.95714286 0.97142857 0.98571429 1 1 1 1 1 1
  arc A9 (-6.8073, -11.0752) -> (-6.1877, -11.4329) centre (0, 0) ccw
  spline S9 degree 5 poles (-6.1877, -11.4329) (-6.183, -11.43) (-6.1735, -11.4241) (-6.1593, -11.4153) (-6.1404, -11.4034) (-6.1169, -11.3885) (-6.0935, -11.3735) (-6.0701, -11.3585) (-6.0469, -11.3433) (-6.0238, -11.3281) (-6.0008, -11.3128) (-5.9779, -11.2974) (-5.9551, -11.2819) (-5.9324, -11.2664) (-5.9098, -11.2507) (-5.8873, -11.235) (-5.8649, -11.2192) (-5.8427, -11.2033) (-5.8205, -11.1873) (-5.7985, -11.1713) (-5.7765, -11.1552) (-5.7547, -11.1389) (-5.733, -11.1226) (-5.7114, -11.1062) (-5.6899, -11.0898) (-5.6685, -11.0732) (-5.6473, -11.0566) (-5.6261, -11.0399) (-5.6051, -11.023) (-5.5842, -11.0062) (-5.5635, -10.9892) (-5.5428, -10.9721) (-5.5223, -10.955) (-5.5019, -10.9377) (-5.4817, -10.9204) (-5.4615, -10.903) (-5.4415, -10.8855) (-5.4216, -10.8679) (-5.4019, -10.8502) (-5.3823, -10.8324) (-5.3628, -10.8146) (-5.3435, -10.7966) (-5.3243, -10.7786) (-5.3053, -10.7605) (-5.2864, -10.7422) (-5.2677, -10.7239) (-5.2491, -10.7055) (-5.2307, -10.687) (-5.2124, -10.6684) (-5.1942, -10.6497) (-5.1763, -10.6309) (-5.1585, -10.612) (-5.1409, -10.593) (-5.1235, -10.5739) (-5.1063, -10.5547) (-5.0892, -10.5353) (-5.0723, -10.5159) (-5.0555, -10.4964) (-5.039, -10.4768) (-5.0226, -10.4571) (-5.0065, -10.4372) (-4.9907, -10.4172) (-4.9751, -10.397) (-4.9599, -10.3767) (-4.9449, -10.3562) (-4.9301, -10.3356) (-4.9155, -10.315) (-4.901, -10.2942) (-4.8867, -10.2734) (-4.8728, -10.2523) (-4.8596, -10.231) (-4.8497, -10.2135) (-4.8427, -10.2002) (-4.8383, -10.1912) (-4.8361, -10.1866) knots -1 -1 -1 -1 -1 -1 -0.98571429 -0.97142857 -0.95714286 -0.94285714 -0.92857143 -0.91428571 -0.9 -0.88571429 -0.87142857 -0.85714286 -0.84285714 -0.82857143 -0.81428571 -0.8 -0.78571429 -0.77142857 -0.75714286 -0.74285714 -0.72857143 -0.71428571 -0.7 -0.68571429 -0.67142857 -0.65714286 -0.64285714 -0.62857143 -0.61428571 -0.6 -0.58571429 -0.57142857 -0.55714286 -0.54285714 -0.52857143 -0.51428571 -0.5 -0.48571429 -0.47142857 -0.45714286 -0.44285714 -0.42857143 -0.41428571 -0.4 -0.38571429 -0.37142857 -0.35714286 -0.34285714 -0.32857143 -0.31428571 -0.3 -0.28571429 -0.27142857 -0.25714286 -0.24285714 -0.22857143 -0.21428571 -0.2 -0.18571429 -0.17142857 -0.15714286 -0.14285714 -0.12857143 -0.11428571 -0.1 -0.08571429 -0.07142857 -0.05714286 -0.04285714 -0.02857143 -0.01428571 0 0 0 0 0 0
  line L13 (-4.8361, -10.1866) -> (-4.6093, -9.7108)
  arc A10 (-4.6093, -9.7108) -> (-3.6073, -10.1259) centre (0, 0) ccw
  line L14 (-3.6073, -10.1259) -> (-3.7834, -10.6227)
  spline S10 degree 5 poles (-3.7834, -10.6227) (-3.7851, -10.6274) (-3.7883, -10.6369) (-3.7928, -10.6513) (-3.7981, -10.6706) (-3.8039, -10.6951) (-3.809, -10.7198) (-3.8136, -10.7446) (-3.818, -10.7695) (-3.8223, -10.7945) (-3.8264, -10.8195) (-3.8302, -10.8446) (-3.8339, -10.8698) (-3.8371, -10.895) (-3.8401, -10.9204) (-3.8427, -10.9458) (-3.8451, -10.9713) (-3.8473, -10.9969) (-3.8492, -11.0225) (-3.851, -11.0482) (-3.8526, -11.0739) (-3.854, -11.0997) (-3.8552, -11.1256) (-3.8562, -11.1514) (-3.857, -11.1774) (-3.8576, -11.2034) (-3.858, -11.2294) (-3.8582, -11.2555) (-3.8583, -11.2816) (-3.8581, -11.3078) (-3.8578, -11.334) (-3.8574, -11.3602) (-3.8567, -11.3865) (-3.8559, -11.4128) (-3.855, -11.4392) (-3.8538, -11.4656) (-3.8525, -11.492) (-3.8511, -11.5184) (-3.8495, -11.5449) (-3.8477, -11.5714) (-3.8458, -11.598) (-3.8437, -11.6246) (-3.8415, -11.6512) (-3.8391, -11.6778) (-3.8365, -11.7045) (-3.8339, -11.7312) (-3.831, -11.7579) (-3.8281, -11.7846) (-3.825, -11.8114) (-3.8217, -11.8382) (-3.8183, -11.865) (-3.8147, -11.8919) (-3.8111, -11.9187) (-3.8072, -11.9456) (-3.8033, -11.9725) (-3.7992, -11.9994) (-3.7949, -12.0264) (-3.7905, -12.0533) (-3.786, -12.0803) (-3.7814, -12.1073) (-3.7766, -12.1343) (-3.7717, -12.1614) (-3.7666, -12.1884) (-3.7614, -12.2155) (-3.7561, -12.2426) (-3.7507, -12.2696) (-3.7451, -12.2968) (-3.7394, -12.3239) (-3.7336, -12.351) (-3.7276, -12.3782) (-3.7215, -12.4053) (-3.7165, -12.4271) (-3.7127, -12.4434) (-3.7102, -12.4543) (-3.7089, -12.4597) knots 0 0 0 0 0 0 0.01428571 0.02857143 0.04285714 0.05714286 0.07142857 0.08571429 0.1 0.11428571 0.12857143 0.14285714 0.15714286 0.17142857 0.18571429 0.2 0.21428571 0.22857143 0.24285714 0.25714286 0.27142857 0.28571429 0.3 0.31428571 0.32857143 0.34285714 0.35714286 0.37142857 0.38571429 0.4 0.41428571 0.42857143 0.44285714 0.45714286 0.47142857 0.48571429 0.5 0.51428571 0.52857143 0.54285714 0.55714286 0.57142857 0.58571429 0.6 0.61428571 0.62857143 0.64285714 0.65714286 0.67142857 0.68571429 0.7 0.71428571 0.72857143 0.74285714 0.75714286 0.77142857 0.78571429 0.8 0.81428571 0.82857143 0.84285714 0.85714286 0.87142857 0.88571429 0.9 0.91428571 0.92857143 0.94285714 0.95714286 0.97142857 0.98571429 1 1 1 1 1 1
  arc A11 (-3.7089, -12.4597) -> (-3.0178, -12.6449) centre (0, 0) ccw
  spline S11 degree 5 poles (-3.0178, -12.6449) (-3.014, -12.6408) (-3.0064, -12.6327) (-2.9949, -12.6204) (-2.9797, -12.6041) (-2.9609, -12.5836) (-2.9421, -12.5631) (-2.9235, -12.5425) (-2.905, -12.5219) (-2.8866, -12.5012) (-2.8684, -12.4804) (-2.8502, -12.4596) (-2.8322, -12.4388) (-2.8143, -12.4179) (-2.7965, -12.3969) (-2.7789, -12.3759) (-2.7614, -12.3549) (-2.744, -12.3338) (-2.7267, -12.3126) (-2.7095, -12.2914) (-2.6925, -12.2701) (-2.6756, -12.2488) (-2.6589, -12.2274) (-2.6423, -12.206) (-2.6258, -12.1846) (-2.6094, -12.163) (-2.5932, -12.1415) (-2.5771, -12.1198) (-2.5612, -12.0982) (-2.5454, -12.0764) (-2.5297, -12.0547) (-2.5142, -12.0328) (-2.4988, -12.011) (-2.4836, -11.989) (-2.4685, -11.967) (-2.4535, -11.945) (-2.4387, -11.9229) (-2.4241, -11.9008) (-2.4096, -11.8786) (-2.3953, -11.8564) (-2.3811, -11.8341) (-2.3671, -11.8118) (-2.3532, -11.7894) (-2.3395, -11.7669) (-2.326, -11.7444) (-2.3126, -11.7219) (-2.2995, -11.6993) (-2.2864, -11.6767) (-2.2736, -11.654) (-2.2609, -11.6312) (-2.2484, -11.6084) (-2.2361, -11.5855) (-2.2241, -11.5626) (-2.2122, -11.5397) (-2.2005, -11.5166) (-2.189, -11.4935) (-2.1777, -11.4704) (-2.1666, -11.4472) (-2.1557, -11.424) (-2.145, -11.4007) (-2.1346, -11.3774) (-2.1244, -11.3539) (-2.1147, -11.3304) (-2.1052, -11.3068) (-2.096, -11.2831) (-2.0871, -11.2594) (-2.0783, -11.2357) (-2.0696, -11.2119) (-2.0612, -11.1881) (-2.0533, -11.1642) (-2.046, -11.1401) (-2.041, -11.1207) (-2.0377, -11.106) (-2.0357, -11.0961) (-2.0348, -11.0912) knots -1 -1 -1 -1 -1 -1 -0.98571429 -0.97142857 -0.95714286 -0.94285714 -0.92857143 -0.91428571 -0.9 -0.88571429 -0.87142857 -0.85714286 -0.84285714 -0.82857143 -0.81428571 -0.8 -0.78571429 -0.77142857 -0.75714286 -0.74285714 -0.72857143 -0.71428571 -0.7 -0.68571429 -0.67142857 -0.65714286 -0.64285714 -0.62857143 -0.61428571 -0.6 -0.58571429 -0.57142857 -0.55714286 -0.54285714 -0.52857143 -0.51428571 -0.5 -0.48571429 -0.47142857 -0.45714286 -0.44285714 -0.42857143 -0.41428571 -0.4 -0.38571429 -0.37142857 -0.35714286 -0.34285714 -0.32857143 -0.31428571 -0.3 -0.28571429 -0.27142857 -0.25714286 -0.24285714 -0.22857143 -0.21428571 -0.2 -0.18571429 -0.17142857 -0.15714286 -0.14285714 -0.12857143 -0.11428571 -0.1 -0.08571429 -0.07142857 -0.05714286 -0.04285714 -0.02857143 -0.01428571 0 0 0 0 0 0
  line L15 (-2.0348, -11.0912) -> (-1.9389, -10.5729)
  arc A12 (-1.9389, -10.5729) -> (-0.8636, -10.7145) centre (0, 0) ccw
  line L16 (-0.8636, -10.7145) -> (-0.9051, -11.2399)
  spline S12 degree 5 poles (-0.9051, -11.2399) (-0.9055, -11.2449) (-0.9062, -11.255) (-0.9068, -11.27) (-0.907, -11.2901) (-0.9062, -11.3152) (-0.9047, -11.3404) (-0.9028, -11.3655) (-0.9006, -11.3907) (-0.8982, -11.416) (-0.8957, -11.4412) (-0.8929, -11.4664) (-0.8899, -11.4917) (-0.8866, -11.5169) (-0.8828, -11.5422) (-0.8788, -11.5674) (-0.8745, -11.5927) (-0.87, -11.6179) (-0.8652, -11.6432) (-0.8603, -11.6685) (-0.8552, -11.6937) (-0.8499, -11.719) (-0.8443, -11.7443) (-0.8386, -11.7695) (-0.8327, -11.7948) (-0.8265, -11.82) (-0.8202, -11.8453) (-0.8136, -11.8706) (-0.8069, -11.8958) (-0.8, -11.921) (-0.7929, -11.9463) (-0.7857, -11.9715) (-0.7783, -11.9967) (-0.7707, -12.0219) (-0.7629, -12.0471) (-0.755, -12.0723) (-0.7469, -12.0975) (-0.7387, -12.1227) (-0.7302, -12.1479) (-0.7217, -12.173) (-0.7129, -12.1982) (-0.7041, -12.2233) (-0.695, -12.2484) (-0.6858, -12.2735) (-0.6765, -12.2986) (-0.667, -12.3237) (-0.6573, -12.3488) (-0.6475, -12.3739) (-0.6376, -12.3989) (-0.6275, -12.424) (-0.6173, -12.449) (-0.6069, -12.474) (-0.5964, -12.499) (-0.5858, -12.5239) (-0.575, -12.5489) (-0.564, -12.5738) (-0.553, -12.5988) (-0.5418, -12.6237) (-0.5304, -12.6486) (-0.5189, -12.6735) (-0.5073, -12.6983) (-0.4956, -12.7232) (-0.4837, -12.748) (-0.4717, -12.7728) (-0.4595, -12.7976) (-0.4473, -12.8223) (-0.4349, -12.8471) (-0.4223, -12.8718) (-0.4097, -12.8965) (-0.3969, -12.9212) (-0.384, -12.9458) (-0.3735, -12.9655) (-0.3657, -12.9803) (-0.3604, -12.9902) (-0.3577, -12.9951) knots 0 0 0 0 0 0 0.01428571 0.02857143 0.04285714 0.05714286 0.07142857 0.08571429 0.1 0.11428571 0.12857143 0.14285714 0.15714286 0.17142857 0.18571429 0.2 0.21428571 0.22857143 0.24285714 0.25714286 0.27142857 0.28571429 0.3 0.31428571 0.32857143 0.34285714 0.35714286 0.37142857 0.38571429 0.4 0.41428571 0.42857143 0.44285714 0.45714286 0.47142857 0.48571429 0.5 0.51428571 0.52857143 0.54285714 0.55714286 0.57142857 0.58571429 0.6 0.61428571 0.62857143 0.64285714 0.65714286 0.67142857 0.68571429 0.7 0.71428571 0.72857143 0.74285714 0.75714286 0.77142857 0.78571429 0.8 0.81428571 0.82857143 0.84285714 0.85714286 0.87142857 0.88571429 0.9 0.91428571 0.92857143 0.94285714 0.95714286 0.97142857 0.98571429 1 1 1 1 1 1
  arc A13 (-0.3577, -12.9951) -> (0.3577, -12.9951) centre (0, 0) ccw
  spline S13 degree 5 poles (0.3577, -12.9951) (0.3604, -12.9902) (0.3657, -12.9803) (0.3735, -12.9655) (0.384, -12.9458) (0.3969, -12.9212) (0.4097, -12.8965) (0.4223, -12.8718) (0.4349, -12.8471) (0.4473, -12.8223) (0.4595, -12.7976) (0.4717, -12.7728) (0.4837, -12.748) (0.4956, -12.7232) (0.5073, -12.6983) (0.5189, -12.6735) (0.5304, -12.6486) (0.5418, -12.6237) (0.553, -12.5988) (0.564, -12.5738) (0.575, -12.5489) (0.5858, -12.5239) (0.5964, -12.499) (0.6069, -12.474) (0.6173, -12.449) (0.6275, -12.424) (0.6376, -12.3989) (0.6475, -12.3739) (0.6573, -12.3488) (0.667, -12.3237) (0.6765, -12.2986) (0.6858, -12.2735) (0.695, -12.2484) (0.7041, -12.2233) (0.7129, -12.1982) (0.7217, -12.173) (0.7302, -12.1479) (0.7387, -12.1227) (0.7469, -12.0975) (0.755, -12.0723) (0.7629, -12.0471) (0.7707, -12.0219) (0.7783, -11.9967) (0.7857, -11.9715) (0.7929, -11.9463) (0.8, -11.921) (0.8069, -11.8958) (0.8136, -11.8706) (0.8202, -11.8453) (0.8265, -11.82) (0.8327, -11.7948) (0.8386, -11.7695) (0.8443, -11.7443) (0.8499, -11.719) (0.8552, -11.6937) (0.8603, -11.6685) (0.8652, -11.6432) (0.87, -11.6179) (0.8745, -11.5927) (0.8788, -11.5674) (0.8828, -11.5422) (0.8866, -11.5169) (0.8899, -11.4917) (0.8929, -11.4664) (0.8957, -11.4412) (0.8982, -11.416) (0.9006, -11.3907) (0.9028, -11.3655) (0.9047, -11.3404) (0.9062, -11.3152) (0.907, -11.2901) (0.9068, -11.27) (0.9062, -11.255) (0.9055, -11.2449) (0.9051, -11.2399) knots -1 -1 -1 -1 -1 -1 -0.98571429 -0.97142857 -0.95714286 -0.94285714 -0.92857143 -0.91428571 -0.9 -0.88571429 -0.87142857 -0.85714286 -0.84285714 -0.82857143 -0.81428571 -0.8 -0.78571429 -0.77142857 -0.75714286 -0.74285714 -0.72857143 -0.71428571 -0.7 -0.68571429 -0.67142857 -0.65714286 -0.64285714 -0.62857143 -0.61428571 -0.6 -0.58571429 -0.57142857 -0.55714286 -0.54285714 -0.52857143 -0.51428571 -0.5 -0.48571429 -0.47142857 -0.45714286 -0.44285714 -0.42857143 -0.41428571 -0.4 -0.38571429 -0.37142857 -0.35714286 -0.34285714 -0.32857143 -0.31428571 -0.3 -0.28571429 -0.27142857 -0.25714286 -0.24285714 -0.22857143 -0.21428571 -0.2 -0.18571429 -0.17142857 -0.15714286 -0.14285714 -0.12857143 -0.11428571 -0.1 -0.08571429 -0.07142857 -0.05714286 -0.04285714 -0.02857143 -0.01428571 0 0 0 0 0 0
  line L17 (0.9051, -11.2399) -> (0.8636, -10.7145)
  arc A14 (0.8636, -10.7145) -> (1.9389, -10.5729) centre (0, 0) ccw
  line L18 (1.9389, -10.5729) -> (2.0348, -11.0912)
  spline S14 degree 5 poles (2.0348, -11.0912) (2.0357, -11.0961) (2.0377, -11.106) (2.041, -11.1207) (2.046, -11.1401) (2.0533, -11.1642) (2.0612, -11.1881) (2.0696, -11.2119) (2.0783, -11.2357) (2.0871, -11.2594) (2.096, -11.2831) (2.1052, -11.3068) (2.1147, -11.3304) (2.1244, -11.3539) (2.1346, -11.3774) (2.145, -11.4007) (2.1557, -11.424) (2.1666, -11.4472) (2.1777, -11.4704) (2.189, -11.4935) (2.2005, -11.5166) (2.2122, -11.5397) (2.2241, -11.5626) (2.2361, -11.5855) (2.2484, -11.6084) (2.2609, -11.6312) (2.2736, -11.654) (2.2864, -11.6767) (2.2995, -11.6993) (2.3126, -11.7219) (2.326, -11.7444) (2.3395, -11.7669) (2.3532, -11.7894) (2.3671, -11.8118) (2.3811, -11.8341) (2.3953, -11.8564) (2.4096, -11.8786) (2.4241, -11.9008) (2.4387, -11.9229) (2.4535, -11.945) (2.4685, -11.967) (2.4836, -11.989) (2.4988, -12.011) (2.5142, -12.0328) (2.5297, -12.0547) (2.5454, -12.0764) (2.5612, -12.0982) (2.5771, -12.1198) (2.5932, -12.1415) (2.6094, -12.163) (2.6258, -12.1846) (2.6423, -12.206) (2.6589, -12.2274) (2.6756, -12.2488) (2.6925, -12.2701) (2.7095, -12.2914) (2.7267, -12.3126) (2.744, -12.3338) (2.7614, -12.3549) (2.7789, -12.3759) (2.7965, -12.3969) (2.8143, -12.4179) (2.8322, -12.4388) (2.8502, -12.4596) (2.8684, -12.4804) (2.8866, -12.5012) (2.905, -12.5219) (2.9235, -12.5425) (2.9421, -12.5631) (2.9609, -12.5836) (2.9797, -12.6041) (2.9949, -12.6204) (3.0064, -12.6327) (3.014, -12.6408) (3.0178, -12.6449) knots 0 0 0 0 0 0 0.01428571 0.02857143 0.04285714 0.05714286 0.07142857 0.08571429 0.1 0.11428571 0.12857143 0.14285714 0.15714286 0.17142857 0.18571429 0.2 0.21428571 0.22857143 0.24285714 0.25714286 0.27142857 0.28571429 0.3 0.31428571 0.32857143 0.34285714 0.35714286 0.37142857 0.38571429 0.4 0.41428571 0.42857143 0.44285714 0.45714286 0.47142857 0.48571429 0.5 0.51428571 0.52857143 0.54285714 0.55714286 0.57142857 0.58571429 0.6 0.61428571 0.62857143 0.64285714 0.65714286 0.67142857 0.68571429 0.7 0.71428571 0.72857143 0.74285714 0.75714286 0.77142857 0.78571429 0.8 0.81428571 0.82857143 0.84285714 0.85714286 0.87142857 0.88571429 0.9 0.91428571 0.92857143 0.94285714 0.95714286 0.97142857 0.98571429 1 1 1 1 1 1
  arc A15 (3.0178, -12.6449) -> (3.7089, -12.4597) centre (0, 0) ccw
  spline S15 degree 5 poles (3.7089, -12.4597) (3.7102, -12.4543) (3.7127, -12.4434) (3.7165, -12.4271) (3.7215, -12.4053) (3.7276, -12.3782) (3.7336, -12.351) (3.7394, -12.3239) (3.7451, -12.2968) (3.7507, -12.2696) (3.7561, -12.2426) (3.7614, -12.2155) (3.7666, -12.1884) (3.7717, -12.1614) (3.7766, -12.1343) (3.7814, -12.1073) (3.786, -12.0803) (3.7905, -12.0533) (3.7949, -12.0264) (3.7992, -11.9994) (3.8033, -11.9725) (3.8072, -11.9456) (3.8111, -11.9187) (3.8147, -11.8919) (3.8183, -11.865) (3.8217, -11.8382) (3.825, -11.8114) (3.8281, -11.7846) (3.831, -11.7579) (3.8339, -11.7312) (3.8365, -11.7045) (3.8391, -11.6778) (3.8415, -11.6512) (3.8437, -11.6246) (3.8458, -11.598) (3.8477, -11.5714) (3.8495, -11.5449) (3.8511, -11.5184) (3.8525, -11.492) (3.8538, -11.4656) (3.855, -11.4392) (3.8559, -11.4128) (3.8567, -11.3865) (3.8574, -11.3602) (3.8578, -11.334) (3.8581, -11.3078) (3.8583, -11.2816) (3.8582, -11.2555) (3.858, -11.2294) (3.8576, -11.2034) (3.857, -11.1774) (3.8562, -11.1514) (3.8552, -11.1256) (3.854, -11.0997) (3.8526, -11.0739) (3.851, -11.0482) (3.8492, -11.0225) (3.8473, -10.9969) (3.8451, -10.9713) (3.8427, -10.9458) (3.8401, -10.9204) (3.8371, -10.895) (3.8339, -10.8698) (3.8302, -10.8446) (3.8264, -10.8195) (3.8223, -10.7945) (3.818, -10.7695) (3.8136, -10.7446) (3.809, -10.7198) (3.8039, -10.6951) (3.7981, -10.6706) (3.7928, -10.6513) (3.7883, -10.6369) (3.7851, -10.6274) (3.7834, -10.6227) knots -1 -1 -1 -1 -1 -1 -0.98571429 -0.97142857 -0.95714286 -0.94285714 -0.92857143 -0.91428571 -0.9 -0.88571429 -0.87142857 -0.85714286 -0.84285714 -0.82857143 -0.81428571 -0.8 -0.78571429 -0.77142857 -0.75714286 -0.74285714 -0.72857143 -0.71428571 -0.7 -0.68571429 -0.67142857 -0.65714286 -0.64285714 -0.62857143 -0.61428571 -0.6 -0.58571429 -0.57142857 -0.55714286 -0.54285714 -0.52857143 -0.51428571 -0.5 -0.48571429 -0.47142857 -0.45714286 -0.44285714 -0.42857143 -0.41428571 -0.4 -0.38571429 -0.37142857 -0.35714286 -0.34285714 -0.32857143 -0.31428571 -0.3 -0.28571429 -0.27142857 -0.25714286 -0.24285714 -0.22857143 -0.21428571 -0.2 -0.18571429 -0.17142857 -0.15714286 -0.14285714 -0.12857143 -0.11428571 -0.1 -0.08571429 -0.07142857 -0.05714286 -0.04285714 -0.02857143 -0.01428571 0 0 0 0 0 0
  line L19 (3.7834, -10.6227) -> (3.6073, -10.1259)
  arc A16 (3.6073, -10.1259) -> (4.6093, -9.7108) centre (0, 0) ccw
  line L20 (4.6093, -9.7108) -> (4.8361, -10.1866)